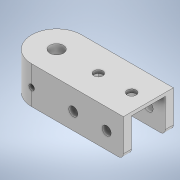
# Autodesk Inventor part: Soporte antebrazo
Saved by Autodesk Inventor 2022 (Build 260153000, 153)
## iProperties
Created: 2022-03-11
Part Number: Soporte antebrazo
Material: Genérico
Document SubType Name: Modeling
Designer: JK
Density: 1 g/cm^3
Appearance: Valor por defecto
Author: JK
Autodesk Inventor part; units mm, degrees
ref_plane "YZ Plane" through (0, 0, 0) normal (1, 0, 0) x (0, 1, 0)
ref_plane "XZ Plane" through (0, 0, 0) normal (0, 1, 0) x (-1, 0, 0)
ref_plane "XY Plane" through (0, 0, 0) normal (0, 0, 1) x (1, 0, 0)
sketch "Boceto1" plane through (0, 0, 0) normal (0, 1, 0) x (-1, 0, 0)
  circle A0 centre (0, 0) radius 4.125
  circle A1 centre (0, 0) radius 15
  dimension "d0" = 8.25
  dimension "d1" = 30
  constraints: 2 centre point, 2 coincident
  measures "d0" diameter of A0
  measures "d1" diameter of A1
extrude "Extrusión1" add sketch "Boceto1" along normal blind 20
sketch "Boceto2" plane through (0, 20, 0) normal (0, 1, 0) x (1, 0, 0)
  circle A0 centre (0, 0) radius 15 projected
  line L0 (0, -15) -> (55, -15)
  line L1 (55, -15) -> (55, 15)
  line L2 (55, 15) -> (0, 15)
  line L3 (0, 15) -> (0, -15)
  line L4 (15, -15) -> (15, 15)
  point P0 (0, 15)
  dimension "d4" = 40
  constraints: 10 end point, 2 horizontal, 2 parallel, 2 perpendicular, 2 point on line, 2 other
  measures "d4" distance between parallel lines of L4 L1
extrude "Extrusión2" add sketch "Boceto2" against normal up to surface (20 mm away) contours L4 L0 A0 | L4 L2 L1 L0 | A0 L2 L4
sketch "Boceto3" plane through (0, 20, 0) normal (0, 1, 0) x (1, 0, 0)
  line L0 (95, -10.15) -> (15, -10.15)
  line L1 (15, -10.15) -> (15, 10.15)
  line L2 (15, 10.15) -> (95, 10.15)
  line L3 (95, 10.15) -> (95, -10.15)
  line L4 (55, -15) -> (55, 15) projected
  line L5 (95, -10.15) -> (15, 10.15) construction
  line L6 (15, -10.15) -> (95, 10.15) construction
  point P0 (0, 0)
  point P1 (55, 0)
  point P2 (55, -10.15)
  point P3 (55, 10.15)
  dimension "d7" = 20.3
  dimension "d8" = 40
  constraints: 12 end point, 3 midpoint, 2 parallel, 1 horizontal, 1 perpendicular
  measures "d7" distance between parallel lines of L0 L2
  measures "d8" distance between parallel lines of L4 L1
extrude "Extrusión3" cut sketch "Boceto3" against normal through all contours L0 L1 L2 L4
fillet "Empalme1" radius 3 4 edges at (55, 20, 12.575) (55, 0, 12.575) (55, 20, -12.575) (55, 0, -12.575)
sketch "Boceto4" plane through (0, 0, 15) normal (0, 0, 1) x (1, 0, 0)
  circle A0 centre (25, 10) radius 2.7
  circle A1 centre (45, 10) radius 2.7
  line L0 (55, 17) -> (55, 3) projected
  line L1 (52, 0) -> (0, 0) projected
  dimension "d12" = 10
  dimension "d13" = 5.4
  dimension "d14" = 10
  dimension "d15" = 20
  constraints: 2 centre point, 1 equal radius, 1 horizontal alignment
  measures "d12" distance from line of L0 A1.centre
  measures "d13" diameter of A1
  measures "d14" distance from line of L1 A1.centre
  measures "d15" distance of A0.centre A1.centre
extrude "Extrusión4" cut sketch "Boceto4" against normal through all
sketch "Boceto5" plane through (0, 0, 15) normal (0, 0, 1) x (1, 0, 0)
  line L0 (0, 0) -> (0, 20) projected
  circle A0 centre (0, 10) radius 1.7
  dimension "d18" = 3.4
  constraints: 1 centre point, 1 midpoint
  measures "d18" diameter of A0
extrude "Extrusión5" cut sketch "Boceto5" against normal blind 15
sketch "Boceto6" plane through (0, 20, 0) normal (0, 1, 0) x (1, 0, 0)
  line L0 (2.85, -6.5) -> (-2.85, -6.5)
  line L1 (-2.85, -6.5) -> (-2.85, -9.5)
  line L2 (-2.85, -9.5) -> (2.85, -9.5)
  line L3 (2.85, -9.5) -> (2.85, -6.5)
  line L4 (2.85, -6.5) -> (-2.85, -9.5) construction
  line L5 (-2.85, -6.5) -> (2.85, -9.5) construction
  point P0 (0, 0)
  point P1 (0, -8)
  point P2 (0, -8)
  point P3 (0, -8)
  dimension "d21" = 3
  dimension "d22" = 5.7
  dimension "d23" = 8
  constraints: 12 end point, 4 midpoint, 2 parallel, 2 vertical alignment, 1 horizontal, 1 perpendicular
  measures "d21" distance of L2.end L0.start
  measures "d22" distance between parallel lines of L3 L1
  measures "d23" distance of point (0, 0) point (0, -8)
extrude "Extrusión6" cut sketch "Boceto6" against normal through all
pattern_circular "Patrón circular1" count 3 over 180 about axis through (0, 0, 0) along (0, -1, 0) of "Extrusión5", "Extrusión6"
sketch "Boceto7" plane through (0, 20, 0) normal (0, 1, 0) x (1, 0, 0)
  line L0 (2.85, 6.5) -> (-2.85, 6.5) projected
  line L1 (-2.85, 6.5) -> (-2.85, 9.5) projected
  line L2 (-2.85, 9.5) -> (2.85, 9.5) projected
  line L3 (2.85, 9.5) -> (2.85, 6.5) projected
  line L4 (-6.5, 2.85) -> (-6.5, -2.85) projected
  line L5 (-6.5, -2.85) -> (-9.5, -2.85) projected
  line L6 (-9.5, -2.85) -> (-9.5, 2.85) projected
  line L7 (-9.5, 2.85) -> (-6.5, 2.85) projected
  line L8 (2.85, -9.5) -> (-2.85, -9.5) projected
  line L9 (-2.85, -9.5) -> (-2.85, -6.5) projected
  line L10 (-2.85, -6.5) -> (2.85, -6.5) projected
  line L11 (2.85, -6.5) -> (2.85, -9.5) projected
  circle A0 centre (0, 0) radius 4.125 projected
  line L12 (52, 15) -> (52, 10.15) projected
  line L13 (52, 15) -> (0, 15) projected
  arc A1 (0, 15) -> (0, -15) centre (0, 0) ccw projected
  line L14 (0, -15) -> (52, -15) projected
  line L15 (52, -10.15) -> (52, -15) projected
  line L16 (52, -10.15) -> (15, -10.15) projected
  line L17 (15, -10.15) -> (15, 10.15) projected
  line L18 (15, 10.15) -> (52, 10.15) projected
extrude "Extrusión7" add sketch "Boceto7" along normal blind 0.3
sketch "Boceto8" plane through (0, 20.3, 0) normal (0, 1, 0) x (1, 0, 0)
  line L0 (15, 10.15) -> (15, -10.15) projected
  line L1 (15, -10.15) -> (52, -10.15) projected
  line L2 (15, 10.15) -> (52, 10.15)
  line L3 (52, 10.15) -> (52, -10.15)
  line L4 (52, -10.15) -> (15, -10.15)
  line L5 (15, -10.15) -> (15, 10.15)
  line L6 (0, -15) -> (52, -15) projected
  line L7 (52, -15) -> (52, -10.15) projected
  line L8 (52, -10.15) -> (15, -10.15) projected
  line L9 (15, -10.15) -> (15, 10.15) projected
  line L10 (15, 10.15) -> (52, 10.15) projected
  line L11 (52, 10.15) -> (52, 15) projected
  line L12 (52, 15) -> (0, 15) projected
  arc A0 (0, 15) -> (0, -15) centre (0, 0) ccw projected
  circle A1 centre (0, 0) radius 4.125 projected
  line L13 (2.85, -9.5) -> (-2.85, -9.5) projected
  line L14 (-2.85, -9.5) -> (-2.85, -6.5) projected
  line L15 (-2.85, -6.5) -> (2.85, -6.5) projected
  line L16 (2.85, -6.5) -> (2.85, -9.5) projected
  line L17 (-6.5, 2.85) -> (-6.5, -2.85) projected
  line L18 (-6.5, -2.85) -> (-9.5, -2.85) projected
  line L19 (-9.5, -2.85) -> (-9.5, 2.85) projected
  line L20 (-9.5, 2.85) -> (-6.5, 2.85) projected
  line L21 (2.85, 6.5) -> (-2.85, 6.5) projected
  line L22 (-2.85, 6.5) -> (-2.85, 9.5) projected
  line L23 (-2.85, 9.5) -> (2.85, 9.5) projected
  line L24 (2.85, 9.5) -> (2.85, 6.5) projected
  line L25 (0, 15) -> (52, 15) projected
  line L26 (55, -15) -> (55, -10.15) projected
  line L27 (52, 15) -> (55, 15)
  line L28 (55, 15) -> (55, -15)
  line L29 (55, -15) -> (52, -15)
  line L30 (52, -15) -> (52, 15)
  constraints: 16 end point, 4 parallel, 2 horizontal, 2 perpendicular
extrude "Extrusión8" add sketch "Boceto8" along normal blind 2
sketch "Boceto9" plane through (55, 3, 10.15) normal (1, 0, 0) x (0, 0, -1)
  line L0 (25.15, 14) -> (25.15, 0) projected
  line L1 (-4.85, 19.3) -> (25.15, 19.3) projected
  line L2 (25.15, 14) -> (20.3, 14)
  line L3 (20.3, 14) -> (20.3, 19.3)
  line L4 (20.3, 19.3) -> (25.15, 19.3)
  line L5 (25.15, 19.3) -> (25.15, 14)
  line L6 (-4.85, 14) -> (-4.85, 0) projected
  line L7 (-4.85, 13.2263) -> (0, 13.2263)
  line L8 (0, 13.2263) -> (0, 19.3)
  line L9 (0, 19.3) -> (-4.85, 19.3)
  line L10 (-4.85, 19.3) -> (-4.85, 13.2263)
  line L11 (0, 0) -> (0, 14) projected
  line L12 (20.3, 14) -> (20.3, 0) projected
  point P0 (10.15, -3)
  point P1 (0, 19.3)
  constraints: 16 end point, 4 parallel, 3 point on line, 2 collinear, 2 horizontal, 2 perpendicular
extrude "Extrusión9" add sketch "Boceto9" against normal blind 5.75
sketch "Boceto10" plane through (0, 22.3, 0) normal (0, 1, 0) x (1, 0, 0)
  line L0 (15, -10.15) -> (15, 10.15) projected
  circle A0 centre (0, 0) radius 4.125 projected
  line L1 (2.85, -9.5) -> (-2.85, -9.5) projected
  line L2 (-2.85, -9.5) -> (-2.85, -6.5) projected
  line L3 (-2.85, -6.5) -> (2.85, -6.5) projected
  line L4 (2.85, -6.5) -> (2.85, -9.5) projected
  line L5 (-6.5, 2.85) -> (-6.5, -2.85) projected
  line L6 (-6.5, -2.85) -> (-9.5, -2.85) projected
  line L7 (-9.5, -2.85) -> (-9.5, 2.85) projected
  line L8 (-9.5, 2.85) -> (-6.5, 2.85) projected
  line L9 (2.85, 6.5) -> (-2.85, 6.5) projected
  line L10 (-2.85, 6.5) -> (-2.85, 9.5) projected
  line L11 (-2.85, 9.5) -> (2.85, 9.5) projected
  line L12 (2.85, 9.5) -> (2.85, 6.5) projected
  line L13 (0, -15) -> (55, -15) projected
  line L14 (55, -15) -> (55, 15) projected
  line L15 (55, 15) -> (0, 15) projected
  arc A1 (0, 15) -> (0, -15) centre (0, 0) ccw projected
extrude "Extrusión10" add sketch "Boceto10" against normal blind 8.8 contours L1 L2 L3 L4 | L5 L6 L7 L8 | L9 L10 L11 L12
sketch "Boceto11" plane through (0, 20.3, 0) normal (0, -1, 0) x (1, 0, 0)
  circle A0 centre (25, 0) radius 2.7
  circle A1 centre (45, 0) radius 2.7
  line L0 (27.7, 10.15) -> (22.3, 10.15) projected
  line L1 (47.7, 10.15) -> (42.3, 10.15) projected
  line L2 (55, 10.15) -> (55, -10.15) projected
  point P0 (0, 0)
  dimension "d37" = 5.4
  dimension "d38" = 10
  dimension "d39" = 20
  constraints: 2 centre point, 1 equal radius
  measures "d37" diameter of A0
  measures "d38" distance from line of L2 A1.centre
  measures "d39" distance of A1.centre A0.centre
extrude "Extrusión11" cut sketch "Boceto11" against normal through all
